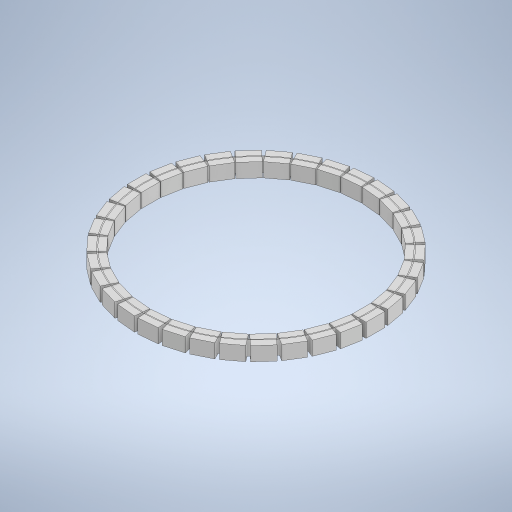
# Autodesk Inventor part: 屋1 物1 柱1
Saved by Autodesk Inventor 2024 (Build 280153000, 153)
## iProperties
Created: 2024-05-23
Part Number: 屋1 物1 柱1
Material: 一般
Document SubType Name: Modeling
Designer: User
Density: 1 g/cm^3
Appearance: 預設
Author: User
Autodesk Inventor part; units mm, degrees
ref_plane "YZ Plane" through (0, 0, 0) normal (1, 0, 0) x (0, 1, 0)
ref_plane "XZ Plane" through (0, 0, 0) normal (0, 1, 0) x (-1, 0, 0)
ref_plane "XY Plane" through (0, 0, 0) normal (0, 0, 1) x (1, 0, 0)
sketch "草圖1" plane through (0, 0, 0) normal (0, 1, 0) x (-1, 0, 0)
  circle A0 centre (0, 0) radius 12
  line L0 (11.25, 1) -> (12.75, 1)
  line L1 (12.75, 1) -> (12.75, -1)
  line L2 (12.75, -1) -> (11.25, -1)
  line L3 (11.25, -1) -> (11.25, 1)
  line L4 (11.25, 1) -> (12.75, -1) construction
  line L5 (12.75, 1) -> (11.25, -1) construction
  line L6 (12.3492, 3.3258) -> (12.7167, 1.3598)
  line L7 (12.7167, 1.3598) -> (11.2422, 1.0842)
  line L8 (11.2422, 1.0842) -> (10.8747, 3.0502)
  line L9 (10.8747, 3.0502) -> (12.3492, 3.3258)
  line L10 (11.5278, 5.5383) -> (12.2503, 3.6734)
  line L11 (12.2503, 3.6734) -> (10.8516, 3.1315)
  line L12 (10.8516, 3.1315) -> (10.1291, 4.9964)
  line L13 (10.1291, 4.9964) -> (11.5278, 5.5383)
  line L14 (10.3138, 7.5622) -> (11.3667, 5.8618)
  line L15 (11.3667, 5.8618) -> (10.0914, 5.0721)
  line L16 (10.0914, 5.0721) -> (9.0385, 6.7726)
  line L17 (9.0385, 6.7726) -> (10.3138, 7.5622)
  line L18 (8.7487, 9.3286) -> (10.0961, 7.8506)
  line L19 (10.0961, 7.8506) -> (8.9875, 6.8401)
  line L20 (8.9875, 6.8401) -> (7.6402, 8.3181)
  line L21 (7.6402, 8.3181) -> (8.7487, 9.3286)
  line L22 (6.8856, 10.7774) -> (8.4816, 9.5721)
  line L23 (8.4816, 9.5721) -> (7.5777, 8.3751)
  line L24 (7.5777, 8.3751) -> (5.9816, 9.5803)
  line L25 (5.9816, 9.5803) -> (6.8856, 10.7774)
  line L26 (4.788, 11.8591) -> (6.5783, 10.9676)
  line L27 (6.5783, 10.9676) -> (5.9097, 9.6248)
  line L28 (5.9097, 9.6248) -> (4.1194, 10.5163)
  line L29 (4.1194, 10.5163) -> (4.788, 11.8591)
  line L30 (2.5274, 12.5369) -> (4.451, 11.9896)
  line L31 (4.451, 11.9896) -> (4.0405, 10.5469)
  line L32 (4.0405, 10.5469) -> (2.1169, 11.0942)
  line L33 (2.1169, 11.0942) -> (2.5274, 12.5369)
  line L34 (0.1807, 12.7879) -> (2.1722, 12.6033)
  line L35 (2.1722, 12.6033) -> (2.0338, 11.1097)
  line L36 (2.0338, 11.1097) -> (0.0423, 11.2943)
  line L37 (0.0423, 11.2943) -> (0.1807, 12.7879)
  line L38 (-2.1722, 12.6033) -> (-0.1807, 12.7879)
  line L39 (-0.1807, 12.7879) -> (-0.0423, 11.2943)
  line L40 (-0.0423, 11.2943) -> (-2.0338, 11.1097)
  line L41 (-2.0338, 11.1097) -> (-2.1722, 12.6033)
  line L42 (-4.451, 11.9896) -> (-2.5274, 12.5369)
  line L43 (-2.5274, 12.5369) -> (-2.1169, 11.0942)
  line L44 (-2.1169, 11.0942) -> (-4.0405, 10.5469)
  line L45 (-4.0405, 10.5469) -> (-4.451, 11.9896)
  line L46 (-6.5783, 10.9676) -> (-4.788, 11.8591)
  line L47 (-4.788, 11.8591) -> (-4.1194, 10.5163)
  line L48 (-4.1194, 10.5163) -> (-5.9097, 9.6248)
  line L49 (-5.9097, 9.6248) -> (-6.5783, 10.9676)
  line L50 (-8.4816, 9.5721) -> (-6.8856, 10.7774)
  line L51 (-6.8856, 10.7774) -> (-5.9816, 9.5803)
  line L52 (-5.9816, 9.5803) -> (-7.5777, 8.3751)
  line L53 (-7.5777, 8.3751) -> (-8.4816, 9.5721)
  line L54 (-10.0961, 7.8506) -> (-8.7487, 9.3286)
  line L55 (-8.7487, 9.3286) -> (-7.6402, 8.3181)
  line L56 (-7.6402, 8.3181) -> (-8.9875, 6.8401)
  line L57 (-8.9875, 6.8401) -> (-10.0961, 7.8506)
  line L58 (-11.3667, 5.8618) -> (-10.3138, 7.5622)
  line L59 (-10.3138, 7.5622) -> (-9.0385, 6.7726)
  line L60 (-9.0385, 6.7726) -> (-10.0914, 5.0721)
  line L61 (-10.0914, 5.0721) -> (-11.3667, 5.8618)
  line L62 (-12.2503, 3.6734) -> (-11.5278, 5.5383)
  line L63 (-11.5278, 5.5383) -> (-10.1291, 4.9964)
  line L64 (-10.1291, 4.9964) -> (-10.8516, 3.1315)
  line L65 (-10.8516, 3.1315) -> (-12.2503, 3.6734)
  line L66 (-12.7167, 1.3598) -> (-12.3492, 3.3258)
  line L67 (-12.3492, 3.3258) -> (-10.8747, 3.0502)
  line L68 (-10.8747, 3.0502) -> (-11.2422, 1.0842)
  line L69 (-11.2422, 1.0842) -> (-12.7167, 1.3598)
  line L70 (-12.75, -1) -> (-12.75, 1)
  line L71 (-12.75, 1) -> (-11.25, 1)
  line L72 (-11.25, 1) -> (-11.25, -1)
  line L73 (-11.25, -1) -> (-12.75, -1)
  line L74 (-12.3492, -3.3258) -> (-12.7167, -1.3598)
  line L75 (-12.7167, -1.3598) -> (-11.2422, -1.0842)
  line L76 (-11.2422, -1.0842) -> (-10.8747, -3.0502)
  line L77 (-10.8747, -3.0502) -> (-12.3492, -3.3258)
  line L78 (-11.5278, -5.5383) -> (-12.2503, -3.6734)
  line L79 (-12.2503, -3.6734) -> (-10.8516, -3.1315)
  line L80 (-10.8516, -3.1315) -> (-10.1291, -4.9964)
  line L81 (-10.1291, -4.9964) -> (-11.5278, -5.5383)
  line L82 (-10.3138, -7.5622) -> (-11.3667, -5.8618)
  line L83 (-11.3667, -5.8618) -> (-10.0914, -5.0721)
  line L84 (-10.0914, -5.0721) -> (-9.0385, -6.7726)
  line L85 (-9.0385, -6.7726) -> (-10.3138, -7.5622)
  line L86 (-8.7487, -9.3286) -> (-10.0961, -7.8506)
  line L87 (-10.0961, -7.8506) -> (-8.9875, -6.8401)
  line L88 (-8.9875, -6.8401) -> (-7.6402, -8.3181)
  line L89 (-7.6402, -8.3181) -> (-8.7487, -9.3286)
  line L90 (-6.8856, -10.7774) -> (-8.4816, -9.5721)
  line L91 (-8.4816, -9.5721) -> (-7.5777, -8.3751)
  line L92 (-7.5777, -8.3751) -> (-5.9816, -9.5803)
  line L93 (-5.9816, -9.5803) -> (-6.8856, -10.7774)
  line L94 (-4.788, -11.8591) -> (-6.5783, -10.9676)
  line L95 (-6.5783, -10.9676) -> (-5.9097, -9.6248)
  line L96 (-5.9097, -9.6248) -> (-4.1194, -10.5163)
  line L97 (-4.1194, -10.5163) -> (-4.788, -11.8591)
  line L98 (-2.5274, -12.5369) -> (-4.451, -11.9896)
  line L99 (-4.451, -11.9896) -> (-4.0405, -10.5469)
  line L100 (-4.0405, -10.5469) -> (-2.1169, -11.0942)
  line L101 (-2.1169, -11.0942) -> (-2.5274, -12.5369)
  line L102 (-0.1807, -12.7879) -> (-2.1722, -12.6033)
  line L103 (-2.1722, -12.6033) -> (-2.0338, -11.1097)
  line L104 (-2.0338, -11.1097) -> (-0.0423, -11.2943)
  line L105 (-0.0423, -11.2943) -> (-0.1807, -12.7879)
  line L106 (2.1722, -12.6033) -> (0.1807, -12.7879)
  line L107 (0.1807, -12.7879) -> (0.0423, -11.2943)
  line L108 (0.0423, -11.2943) -> (2.0338, -11.1097)
  line L109 (2.0338, -11.1097) -> (2.1722, -12.6033)
  line L110 (4.451, -11.9896) -> (2.5274, -12.5369)
  line L111 (2.5274, -12.5369) -> (2.1169, -11.0942)
  line L112 (2.1169, -11.0942) -> (4.0405, -10.5469)
  line L113 (4.0405, -10.5469) -> (4.451, -11.9896)
  line L114 (6.5783, -10.9676) -> (4.788, -11.8591)
  line L115 (4.788, -11.8591) -> (4.1194, -10.5163)
  line L116 (4.1194, -10.5163) -> (5.9097, -9.6248)
  line L117 (5.9097, -9.6248) -> (6.5783, -10.9676)
  line L118 (8.4816, -9.5721) -> (6.8856, -10.7774)
  line L119 (6.8856, -10.7774) -> (5.9816, -9.5803)
  line L120 (5.9816, -9.5803) -> (7.5777, -8.3751)
  line L121 (7.5777, -8.3751) -> (8.4816, -9.5721)
  line L122 (10.0961, -7.8506) -> (8.7487, -9.3286)
  line L123 (8.7487, -9.3286) -> (7.6402, -8.3181)
  line L124 (7.6402, -8.3181) -> (8.9875, -6.8401)
  line L125 (8.9875, -6.8401) -> (10.0961, -7.8506)
  line L126 (11.3667, -5.8618) -> (10.3138, -7.5622)
  line L127 (10.3138, -7.5622) -> (9.0385, -6.7726)
  line L128 (9.0385, -6.7726) -> (10.0914, -5.0721)
  line L129 (10.0914, -5.0721) -> (11.3667, -5.8618)
  line L130 (12.2503, -3.6734) -> (11.5278, -5.5383)
  line L131 (11.5278, -5.5383) -> (10.1291, -4.9964)
  line L132 (10.1291, -4.9964) -> (10.8516, -3.1315)
  line L133 (10.8516, -3.1315) -> (12.2503, -3.6734)
  line L134 (12.7167, -1.3598) -> (12.3492, -3.3258)
  line L135 (12.3492, -3.3258) -> (10.8747, -3.0502)
  line L136 (10.8747, -3.0502) -> (11.2422, -1.0842)
  line L137 (11.2422, -1.0842) -> (12.7167, -1.3598)
  point P0 (12, 0)
  dimension "d0" = 24
  dimension "d1" = 1.5
  dimension "d2" = 2
  dimension "d5" = 360
  constraints: 276 end point, 2 midpoint, 2 parallel, 1 coincident, 1 horizontal, 1 horizontal alignment, 1 perpendicular, 275 other
  measures "d1" distance of L1.end L2.end
  measures "d2" distance of L0.end L1.end
extrude "擠出1" add sketch "草圖1" along normal blind 1.5 contours A0 L2 L3 L0 | A0 L0 L1 L2 | L7 L8 L9 A0 | A0 L9 L6 L7 | L137 L134 L135 A0 | A0 L135 L136 L137 | L11 L12 L13 A0 | A0 L13 L10 L11 | L133 L130 L131 A0 | A0 L131 L132 L133 | L15 L16 L17 A0 | A0 L17 L14 L15 | L129 L126 L127 A0 | A0 L127 L128 L129 | L19 L20 L21 A0 | A0 L21 L18 L19 | L125 L122 L123 A0 | A0 L123 L124 L125 | L23 L24 L25 A0 | A0 L25 L22 L23 | L121 L118 L119 A0 | A0 L119 L120 L121 | L27 L28 L29 A0 | A0 L29 L26 L27 | L117 L114 L115 A0 | A0 L115 L116 L117 | L31 L32 L33 A0 | A0 L33 L30 L31 | L113 L110 L111 A0 | A0 L111 L112 L113 | L35 L36 L37 A0 | A0 L37 L34 L35 | L109 L106 L107 A0 | A0 L107 L108 L109 | L39 L40 L41 A0 | A0 L41 L38 L39 | L105 L102 L103 A0 | A0 L103 L104 L105 | L43 L44 L45 A0 | A0 L45 L42 L43 | L101 L98 L99 A0 | A0 L99 L100 L101 | L47 L48 L49 A0 | A0 L49 L46 L47 | L97 L94 L95 A0 | A0 L95 L96 L97 | L51 L52 L53 A0 | A0 L53 L50 L51 | L93 L90 L91 A0 | A0 L91 L92 L93 | L55 L56 L57 A0 | A0 L57 L54 L55 | L89 L86 L87 A0 | A0 L87 L88 L89 | L59 L60 L61 A0 | A0 L61 L58 L59 | L85 L82 L83 A0 | A0 L83 L84 L85 | L63 L64 L65 A0 | A0 L65 L62 L63 | L81 L78 L79 A0 | A0 L79 L80 L81 | L67 L68 L69 A0 | A0 L69 L66 L67 | L77 L74 L75 A0 | A0 L75 L76 L77 | L71 L72 L73 A0 | A0 L73 L70 L71
sketch "草圖2" plane through (0, 0, 0) normal (0, 1, 0) x (-1, 0, 0)
  circle A0 centre (0, 0) radius 12.05
  circle A1 centre (0, 0) radius 11.95
  dimension "d9" = 24.1
  dimension "d10" = 23.9
  constraints: 2 centre point, 2 coincident
  measures "d9" diameter of A0
  measures "d10" diameter of A1
extrude "擠出2" add sketch "草圖2" along normal blind 1.5 separate body
